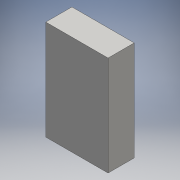
# Autodesk Inventor part: power supply
Saved by Autodesk Inventor 2016 (Build 200138000, 138)
## iProperties
Created: 2017-06-06
Part Number: power supply
Material: Generic
Document SubType Name: Modeling
Designer: fabio-note
Density: 1 g/cm^3
Appearance: Default
Author: fabio-note
Autodesk Inventor part; units mm, degrees
ref_plane "YZ Plane" through (0, 0, 0) normal (1, 0, 0) x (0, 1, 0)
ref_plane "XZ Plane" through (0, 0, 0) normal (0, 1, 0) x (-1, 0, 0)
ref_plane "XY Plane" through (0, 0, 0) normal (0, 0, 1) x (1, 0, 0)
sketch "Sketch1" plane through (0, 0, 0) normal (0, 1, 0) x (-1, 0, 0)
  line L0 (50, 80) -> (-50, 80)
  line L1 (-50, 80) -> (-50, -80)
  line L2 (-50, -80) -> (50, -80)
  line L3 (50, -80) -> (50, 80)
  point P0 (0, 0)
  point P1 (0, -80)
  point P2 (50, 0)
  dimension "d0" = 100
  dimension "d1" = 160
  constraints: 8 end point, 2 midpoint, 2 parallel, 1 horizontal, 1 horizontal alignment, 1 perpendicular, 1 vertical alignment
  measures "d0" distance of L2.end L1.end
  measures "d1" distance between parallel lines of L0 L2
extrude "Extrusion1" add sketch "Sketch1" along normal blind 42
body "Solid1"
